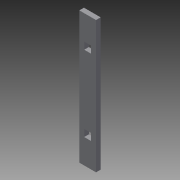
# Autodesk Inventor part: HopperSupportRod_v2
Saved by Autodesk Inventor 2013 (Build 170138000, 138)
## iProperties
Created: 2013-01-17
Part Number: HopperSupportRod_v2
Material: Generic
Document SubType Name: Modeling
Designer: twsass
Density: 1 g/cm^3
Author: twsass
Autodesk Inventor part; units mm, degrees
ref_plane "YZ Plane" through (0, 0, 0) normal (1, 0, 0) x (0, 1, 0)
ref_plane "XZ Plane" through (0, 0, 0) normal (0, 1, 0) x (-1, 0, 0)
ref_plane "XY Plane" through (0, 0, 0) normal (0, 0, 1) x (1, 0, 0)
sketch "Sketch1" plane through (0, 0, 0) normal (0, 0, 1) x (1, 0, 0)
  line L0 (0, 0) -> (22.86, 0)
  line L1 (22.86, 0) -> (22.86, 180.086)
  line L2 (22.86, 180.086) -> (0, 180.086)
  line L3 (0, 180.086) -> (0, 0)
  line L4 (0, 90.043) -> (22.86, 90.043) construction
  line L5 (11.43, 146.431) -> (16.1925, 146.431)
  line L6 (16.1925, 146.431) -> (16.1925, 136.906)
  line L7 (16.1925, 136.906) -> (6.6675, 136.906)
  line L8 (6.6675, 136.906) -> (6.6675, 146.431)
  line L9 (6.6675, 146.431) -> (11.43, 146.431)
  line L10 (11.43, 33.655) -> (16.1925, 33.655)
  line L11 (16.1925, 33.655) -> (16.1925, 43.18)
  line L12 (16.1925, 43.18) -> (6.6675, 43.18)
  line L13 (6.6675, 43.18) -> (6.6675, 33.655)
  line L14 (6.6675, 33.655) -> (11.43, 33.655)
  dimension "d0" = 22.86
  dimension "d1" = 180.086
  dimension "d13" = 4.7625
  dimension "d14" = 9.525
  dimension "d15" = 9.525
  dimension "d16" = 33.655
  dimension "d17" = 6.6675
  constraints: 30 end point, 5 perpendicular, 5 symmetric about line, 2 midpoint, 2 parallel, 2 point on line, 1 collinear, 1 horizontal
  measures "d0" distance of L0.start L0.end
  measures "d1" distance of L0.end L1.end
  measures "d13" distance of L5.start L5.end
  measures "d14" distance of L5.end L6.end
  measures "d15" distance of L6.end L7.end
  measures "d16" distance between parallel lines of L2 L9
  measures "d17" distance between parallel lines of L1 L6
extrude "Extrusion2" add sketch "Sketch1" along normal blind 6.35
body "Solid2"
